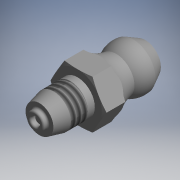
# Autodesk Inventor part: DIN-71412 A M5x0.8/SW7
Saved by Autodesk Inventor 2017.3 (Build 213256000, 256)
## iProperties
Part Number: DIN-71412 A M5x0.8/SW7
Material: Generic
Catalog Web Link: www.cadenas.de
Description: DIN-71412 A-Lubricating nipples; cone type, form A
Vendor: FESTO
Document SubType Name: Modeling
Designer: partserver
Manufacturer: FESTO
Mass: 0.422146 g
Surface Area: 3.53363 cm^2
Volume: 0.422146 cm^3
Density: 1 g/cm^3
Appearance: PSOLRGB-175-175-175
Category: PARTsolutions
Company: FESTO
Title: Kegelschmiernippel DIN 71412 A M5x0.8/SW7
Author: Cadenas PARTsolutions
Comments: Lubricating nipples; cone type, form A
PSOL_IDENT_0: {$CADENAS_DATA\23d-libs\festo\zyl_zubeh\din_71412\din_71412_form_a.prj},224 {M=Nenngewinde},{VTYP=3D
PSOL_IDENT_1: },{NB=DIN-71412 A M5x0.8/SW7},{LINA=Kegelschmiernippel DIN 71412 A M5x0.8/SW7},{NN=DIN-71412 A},{DAT
PSOL_IDENT_2: E=02.07.2015 11:36:46},{GEOMDATE=02.07.2015 11:36:00},{VERSION=},{LINEID=80},{WBVAR=},{WBNUMERIC=}
PSOL_IDENT_3: {NB=DIN-71412 A M5x0.8/SW7},{LINA=Kegelschmiernippel DIN 71412 A M5x0.8/SW7},{KT=DUMMY},{IDNR=},{D=M
PSOL_IDENT_4: 5},{D1=5.000},{P=0.800},{DK=4.020},{S=7.000},{NENN=A M5x0.8/SW7}
NB: DIN-71412 A M5x0.8/SW7
NN: DIN-71412 A
NT: Lubricating nipples; cone type, form A
NBSYN: DIN-71412 $NENN.
LINA: Kegelschmiernippel DIN 71412 A M5x0.8/SW7
CATALOG: Festo
ROWDESC: A M5x0.8/SW7
OFFICIAL_STANDARD_NUMBERS: DIN 71412
D: M5
S: 7
SUPPLIER: FESTO
ARTICLENO: DIN-71412 A M5x0.8/SW7
BOMINFO: Kegelschmiernippel DIN 71412 A M5x0.8/SW7
CREATOR: CADENAS GmbH
Autodesk Inventor part; units mm, degrees
sketch "Sketch_1" plane through (0, 0, 0) normal (0, 0, 1) x (1, 0, 0)
  line L0 (0, -6.2) -> (0, 10.8)
  arc A0 (0.75, 9.5761) -> (0, 9.7048) centre (0, 7.4548) ccw
  line L1 (0.75, 9.5761) -> (0.75, 9.8)
  line L2 (0.75, 9.8) -> (2.25, 9.8)
  line L3 (2.25, 9.8) -> (3.1941, 8.0548)
  arc A1 (2.65, 5.5733) -> (3.1941, 8.0548) centre (0, 7.4548) ccw
  arc A2 (2.65, 5.5733) -> (3.7238, 2.94) centre (8.8225, 6.5548) ccw
  line L4 (3.7238, 2.94) -> (9.0981, 1.5)
  line L5 (9.0981, 1.5) -> (3.5, 0)
  line L6 (3.5, 0) -> (2.5, 0)
  line L7 (2.5, 0) -> (2.5, -3.5)
  line L8 (2.5, -3.5) -> (2.0095, -5.5)
  line L9 (2.0095, -5.5) -> (1.5, -5.5)
  arc A3 (1.5, -5.5) -> (1.25, -5.75) centre (1.5, -5.75) ccw
  line L10 (1.25, -5.75) -> (1.25, -5.95)
  arc A4 (1, -6.2) -> (1.25, -5.95) centre (1, -5.95) ccw
  line L11 (1, -6.2) -> (0.875, -6.2)
  arc A5 (0.625, -5.95) -> (0.875, -6.2) centre (0.875, -5.95) ccw
  line L12 (0.625, -5.95) -> (0.625, -5.5)
  line L13 (0.625, -5.5) -> (0, -5.5)
  line L14 (0, -5.5) -> (0, 9.7048)
  constraints: 30 end point, 12 point on circle, 6 centre point
revolve "Revolution1" add sketch "Sketch_1" angle 360 about axis through (0, -6.2, 0) along (0, 1, 0)
thread "Thread1" size "M5x0.8" class "6g" standard "ISO Metric profile" length 2.5
sketch "Sketch_2" plane through (0, 0, 0) normal (0, 1, 0) x (-1, 0, 0)
  line L0 (14, -14) -> (14, 14)
  line L1 (14, 14) -> (-14, 14)
  line L2 (-14, 14) -> (-14, -14)
  line L3 (-14, -14) -> (14, -14)
  line L4 (4.0415, 0) -> (2.0207, 3.5)
  line L5 (2.0207, 3.5) -> (-2.0207, 3.5)
  line L6 (-2.0207, 3.5) -> (-4.0415, 0)
  line L7 (-4.0415, 0) -> (-2.0207, -3.5)
  line L8 (-2.0207, -3.5) -> (2.0207, -3.5)
  line L9 (2.0207, -3.5) -> (4.0415, 0)
  constraints: 20 end point
extrude "Extrusion1" cut sketch "Sketch_2" along normal blind 5
ref_plane "ANBAU_XY" through (0, 0, 0) normal (0, 1, 0) x (1, 0, 0)
ref_plane "ANBAU_YZ" through (0, 0, 0) normal (1, 0, 0) x (0, 0, -1)
ref_plane "ANBAU_ZX" through (0, 0, 0) normal (0, 0, -1) x (0, 1, 0)
body "Solid1"
